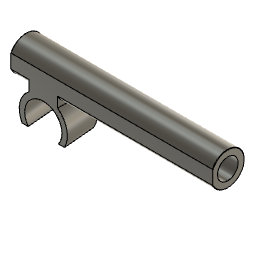
Führung (Autodesk Fusion 360 design; units mm, degrees)
Autodesk Fusion 360 part; units mm, degrees
sketch "Sketch1" plane through (0, 0, 0) normal (1, 0, 0) x (0, 1, 0)
  circle A0 centre (0, 0) radius 3.4288
  circle A1 centre (0, 0) radius 5.5232
  constraint coincident A0.centre A1.centre
extrude "Extrude1" add sketch "Sketch1" along normal blind 55 makes body 1
sketch "Sketch3" plane through (0, 0, 0) normal (0, 1, 0) x (1, 0, 0)
  arc A0 (-6, 20) -> (4, 20) centre (-1, 16.3988) ccw
  arc A1 (-8, 20) -> (6, 20) centre (-1, 16.2604) ccw
  line L0 (-8, 20) -> (-6, 20)
  line L1 (4, 20) -> (6, 20)
  constraint horizontal L0
  constraint parallel L0 L1
extrude "Extrude3" add sketch "Sketch3" along normal blind 10 separate body makes body 2
move_face "MoveFace1" to x (1, 0, 0) y (0, 1, 0) z (0, 0, 1) at (-11.8961, 5.0156, -4.5895) 3 faces at (18.3333, 5.4957, -0.5499) (0, 4.7917, -0.4447) (18.3333, 3.4118, -0.3414) on bodies 1
move_body "Move2" bodies 2 to x (0.996195, 0.087156, 0) y (-0.087156, 0.996195, 0) z (0, 0, 1) at (-0.0344, -0.3202, 0)
move_body "Move3" bodies 2 to x (1, 0, 0) y (0, 1, 0) z (0, 0, 1) at (-0.0936, 0.5352, -0.5148)
combine "Combine2" operation add target body 1 tool bodies 2
fillet "Fillet9" radius 0.1 1 edges at (55, -0.1338, -6.5867) on bodies 1
fillet "Fillet12" radius 0.1 1 edges at (-11.8961, -0.1338, -6.5867) on bodies 1
extrude "Extrude5" add 1 faces at (1.3577, 0.3449, -9.9317) along direction (0.087156, -0.996195, 0) blind 6 on bodies 1 bodies 1
sketch "Sketch6" plane through (0, 0, 0) normal (0, 1, 0) x (1, 0, 0)
  line L0 (-22, -13) -> (64, -13)
  line L1 (64, -13) -> (64, 24)
  line L2 (64, 24) -> (-22, 24)
  line L3 (-22, 24) -> (-22, -13)
  constraint horizontal L0
  constraint vertical L1
  constraint horizontal L2
  constraint vertical L3
extrude "Extrude6" cut sketch "Sketch6" against normal blind 14 bodies 1
sketch "Sketch7" plane through (0, 0, 0) normal (0, -1, 0) x (1, 0, 0)
  ellipse E0 centre (-1.113, -16.7752) end of major axis (-9.0796, -16.7752) minor radius 7.9363 (5.9137, -20.5148) -> (-8.1397, -20.5148) ccw
  line L0 (-8.1397, -20.5148) -> (-6.1321, -20.5148)
  ellipse E1 centre (-1.113, -16.9137) end of major axis (-7.2984, -16.9137) minor radius 6.1618 (3.9061, -20.5148) -> (-6.1321, -20.5148) ccw
  line L1 (3.9061, -20.5148) -> (5.9137, -20.5148)
  line L2 (-5.8366, -5.5777) -> (3.6106, -5.5777)
  line L3 (3.6106, -5.5777) -> (3.6106, -10.3845)
  line L4 (3.6106, -10.3845) -> (-5.8366, -10.3845)
  line L5 (-5.8366, -10.3845) -> (-5.8366, -5.5777)
  constraint horizontal L2
  constraint vertical L3
  constraint horizontal L4
  constraint vertical L5
  constraint coincident E0 L4.end
  constraint coincident E0 L3.end
extrude "Extrude7" add sketch "Sketch7" against normal blind 5 contours E0 L4 | E0 L2 L3 L5 bodies 1
sketch "Sketch8" plane through (-11.8961, 0, 0) normal (-1, 0, 0) x (0, -1, 0)
  line L0 (0, -6.6522) -> (0, -2.5268)
  arc A0 (0, -2.5268) -> (0, -6.6522) centre (-5.0156, -4.5895) ccw
  circle A1 centre (-5.0156, -4.5895) radius 3.4288
  circle A2 centre (-5.0156, -4.5895) radius 3.4288
  constraint concentric A0 A2
extrude "Extrude8" cut sketch "Sketch8" against normal blind 115 contours A1 A2 bodies 1
